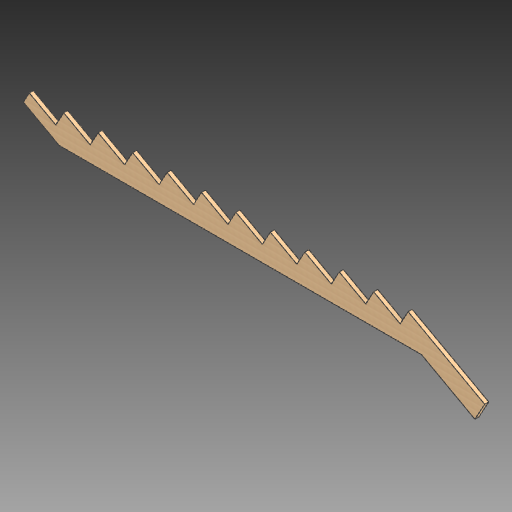
# Autodesk Inventor part: Косоур-1
Saved by Autodesk Inventor 2019 (Build 230136000, 136)
## iProperties
Created: 2018-10-10
Part Number: Косоур-1
Material: Ясень
Document SubType Name: Modeling
Designer: Андреев Н.Л.
Density: 0.641 g/cm^3
Appearance: Дверь — ясень
ШИРИНА: 300
ДЛИНА: 4533
ТОЛЩВЫС: 40
Author: Андреев Н.Л.
Autodesk Inventor part; units mm, degrees
ref_plane "YZ Plane" through (0, 0, 0) normal (1, 0, 0) x (0, 1, 0)
ref_plane "XZ Plane" through (0, 0, 0) normal (0, 1, 0) x (-1, 0, 0)
ref_plane "XY Plane" through (0, 0, 0) normal (0, 0, 1) x (1, 0, 0)
sketch "Эскиз1" plane through (0, 0, 0) normal (0, 1, 0) x (-1, 0, 0)
  line L0 (-351.6863, -300) -> (-3912.4146, -300)
  line L1 (-3780.9356, 0) -> (-397.2026, 0)
  line L2 (0, -107.4494) -> (-351.6863, -300)
  line L3 (0, -107.4494) -> (-58.8293, 0)
  line L4 (-58.8293, 0) -> (-319.1637, -142.5349)
  line L5 (-319.1637, -142.5349) -> (-397.2026, 0)
  line L6 (-397.2026, 0) -> (-657.537, -142.5349) construction
  line L7 (-657.537, -142.5349) -> (-319.1637, -142.5349) construction
  line L8 (-3780.9356, 0) -> (-4532.9935, -411.7568)
  line L9 (-4532.9935, -411.7568) -> (-4436.9457, -587.1843)
  line L10 (-4436.9457, -587.1843) -> (-3912.4146, -300)
  point P0 (0, 0)
  dimension "d0" = 300
  dimension "d4" = 162.5
  dimension "d5" = 296.8
  dimension "d6" = 338.3733
  dimension "Выс1" = 122.5
  dimension "Длина1" = 296.8
  dimension "Выс2" = 200
  dimension "Длина" = 3383.733
  dimension "Длина2" = 857.4
  constraints: 22 end point, 4 perpendicular, 3 parallel, 2 horizontal, 1 point on line, 1 vertical alignment
  measures "d0" distance between parallel lines of L0 L1
  measures "d4" distance of L4.end L1.end
  measures "d5" distance of L1.end L6.end
  measures "d6" distance of L6.end L4.end
  measures "Выс1" distance of L2.start L3.end
  measures "Длина1" distance of L3.end L4.end
  measures "Выс2" distance of L8.end L9.end
  measures "Длина" distance of L1.start L1.end
  measures "Длина2" distance of L1.start L8.end
extrude "Выдавливание1" add sketch "Эскиз1" along normal blind 40
sketch "Эскиз2" plane through (0, 0, 0) normal (0, 1, 0) x (-1, 0, 0)
  line L0 (-397.2026, 0) -> (-3780.9356, 0) construction
  line L1 (-3780.9356, 0) -> (-4532.9935, -411.7568) construction
  line L2 (-4532.9935, -411.7568) -> (-4436.9457, -587.1843) construction
  line L3 (-4436.9457, -587.1843) -> (-3912.4146, -300) construction
  line L4 (-3912.4146, -300) -> (-351.6863, -300) construction
  line L5 (-351.6863, -300) -> (0, -107.4494) construction
  line L6 (0, -107.4494) -> (-58.8293, 0) construction
  line L7 (-58.8293, 0) -> (-319.1637, -142.5349) construction
  line L8 (-319.1637, -142.5349) -> (-397.2026, 0) construction
  line L9 (-397.2026, 0) -> (-657.537, -142.5349)
  line L10 (-657.537, -142.5349) -> (-735.5759, 0)
  line L11 (-735.5759, 0) -> (-397.2026, 0)
  point P0 (0, 0)
  dimension "d12" = 338.3733
  constraints: 6 end point, 1 collinear, 1 horizontal alignment, 1 perpendicular, 1 point on line
  measures "d12" distance of L10.end L0.start
extrude "Выдавливание2" cut sketch "Эскиз2" along normal through all
pattern_linear "Прямоуг.массив1" count 10 spacing 338.3733 along (1, 0, 0) of "Выдавливание2"
equation "\"d0\" = пШирКосоура"
equation "\"d4\" = пПодъем"
equation "\"d5\" = пХод"
equation "\"d6\" = пДиаг"
equation "\"Выс1\" = пПодъем - пТолПроступи"
equation "\"Длина1\" = пХод"
equation "\"Выс2\" = 0.666667 * пШирКосоура"
equation "\"Длина2\" = -пСвес + пДлПроступи + пОтступОтСтен - пТолПодступенка"
equation "\"d2\" = пТолКосоура"
equation "\"d12\" = пДиаг"
equation "\"d13\" = пТолКосоура"
equation "\"d17\" = пДиаг"
equation "\"пДлПроступи\" = 900"
equation "\"пПодъем\" = 162.5"
equation "\"пХод\" = 296.8"
equation "\"пЭффШаг\" = 621.8"
equation "\"пСвес\" = 30.2"
equation "\"пТолПроступи\" = 40"
equation "\"пТолКосоура\" = 40"
equation "\"пШирКосоура\" = 300"
equation "\"пОтступСтен\" = 5"
equation "\"пДиаг\" = 338.3733"
equation "\"пШирПроступи\" = 327"
equation "\"пТолПодступенка\" = 17.4"
equation "\"пГлубПаза\" = 12"
equation "\"пОтступОтСтен\" = 5"
equation "\"пТолПричала\" = 17.4"
equation "\"ДЛИНА\" = 4532.99348"
